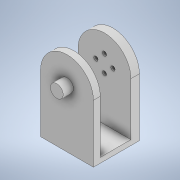
# Autodesk Inventor part: Base_Mount
Saved by Autodesk Inventor 2022 (Build 260153000, 153)
## iProperties
Created: 2022-04-03
Part Number: Base_Mount
Material: Generic
Document SubType Name: Modeling
Designer: Mlees
Density: 1 g/cm^3
Appearance: Default
Author: Mlees
Autodesk Inventor part; units mm, degrees
ref_plane "YZ Plane" through (0, 0, 0) normal (1, 0, 0) x (0, 1, 0)
ref_plane "XZ Plane" through (0, 0, 0) normal (0, 1, 0) x (-1, 0, 0)
ref_plane "XY Plane" through (0, 0, 0) normal (0, 0, 1) x (1, 0, 0)
sketch "Sketch1" plane through (0, 0, 0) normal (0, 0, 1) x (1, 0, 0)
  arc A0 (15.5, 0) -> (-15.5, 0) centre (0, 0) ccw
  line L0 (-15.5, 0) -> (-15.5, -34)
  line L1 (-15.5, -34) -> (15.5, -34)
  line L2 (15.5, -34) -> (15.5, 0)
  circle A1 centre (0, 5) radius 1.25
  circle A2 centre (-5, 0) radius 1.25
  circle A3 centre (0, -5) radius 1.25
  circle A4 centre (5, 0) radius 1.25
  dimension "d0" = 31
  dimension "d1" = 34
  dimension "d3" = 2.5
  dimension "d6" = 360
  constraints: 6 end point, 5 centre point, 2 point on circle, 2 tangent, 1 coincident, 1 perpendicular, 1 vertical, 9 other
  measures "d0" diameter of A0
  measures "d1" distance of L0.start L0.end
  measures "d3" diameter of A1
extrude "Extrusion1" add sketch "Sketch1" along normal blind 5
sketch "Sketch2" plane through (0, 0, 5) normal (0, 0, 1) x (1, 0, 0)
  line L0 (-15.5, -34) -> (15.5, -34) projected
  line L1 (15.5, -34) -> (15.5, 0) projected
  line L2 (-15.5, -34) -> (15.5, -34)
  line L3 (15.5, -34) -> (15.5, -31)
  line L4 (15.5, -31) -> (-15.5, -31)
  line L5 (-15.5, -31) -> (-15.5, -34)
  point P0 (0, 0)
  dimension "d10" = 3
  constraints: 8 end point, 2 parallel, 1 horizontal, 1 perpendicular, 1 point on line
  measures "d10" distance of L3.end L2.end
extrude "Extrusion2" add sketch "Sketch2" along normal blind 22
sketch "Sketch3" plane through (0, 0, 27) normal (0, 0, 1) x (1, 0, 0)
  line L0 (15.5, -31) -> (-15.5, -31) projected
  line L1 (15.5, -34) -> (15.5, 0) projected
  line L2 (15.5, -31) -> (15.5, 0)
  line L3 (-15.5, 0) -> (-15.5, -31) projected
  line L4 (-15.5, 0) -> (-15.5, -31)
  line L5 (-15.5, -31) -> (15.5, -31)
  arc A0 (15.5, 0) -> (-15.5, 0) centre (0, 0) ccw
  point P0 (0, 0)
  constraints: 6 end point, 2 point on circle, 2 tangent, 1 centre point, 1 collinear, 1 perpendicular, 1 vertical
extrude "Extrusion3" add sketch "Sketch3" against normal blind 4
sketch "Sketch4" plane through (0, 0, 0) normal (0, 0, -1) x (-1, 0, 0)
  circle A0 centre (0, 0) radius 3.75
  dimension "d15" = 7.5
  constraints: 1 centre point, 1 coincident
  measures "d15" diameter of A0
extrude "Extrusion4" add sketch "Sketch4" along normal blind 6
sketch "Sketch5" plane through (0, 0, 27) normal (0, 0, 1) x (1, 0, 0)
  circle A0 centre (0, 0) radius 3.75
  dimension "d20" = 7.5
  constraints: 1 centre point, 1 coincident
  measures "d20" diameter of A0
extrude "Extrusion5" add sketch "Sketch5" along normal blind 6
body "Solid1"
